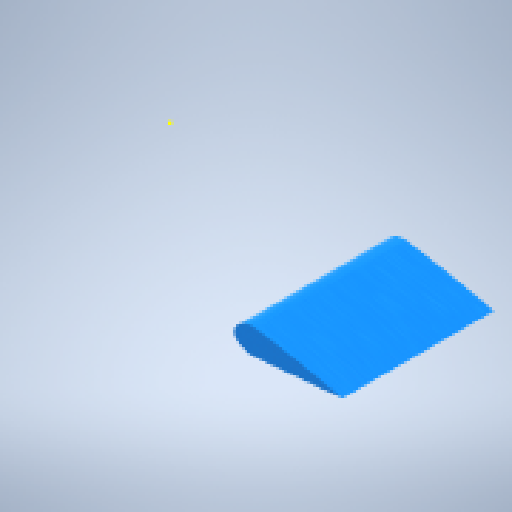
# Autodesk Inventor part: AIL outboard outer foam assembly
Saved by Autodesk Inventor 2025.2 (Build 292293000, 293)
## iProperties
Created: 2024-11-18
Part Number: AIL outboard outer foam assembly
Material: Polyurethane Foam
Document SubType Name: Modeling
Designer: thoma
Density: 0.032 g/cm^3
Appearance: Coarse Textured - Umber
Author: thoma
Autodesk Inventor part; units mm, degrees
ref_plane "YZ Plane" through (0, 0, 0) normal (1, 0, 0) x (0, 1, 0)
ref_plane "XZ Plane" through (0, 0, 0) normal (0, 1, 0) x (-1, 0, 0)
ref_plane "XY Plane" through (0, 0, 0) normal (0, 0, 1) x (1, 0, 0)
sketch "Sketch1" plane through (0, 0, 0) normal (0, 0, 1) x (1, 0, 0)
  spline S0 degree 5 poles (217.3654, -7.5638) (217.3859, -7.562) (219.4778, -7.3868) (223.5726, -7.0416) (229.5629, -6.5311) (237.2988, -5.8637) (246.5067, -5.0508) (255.1715, -4.2808) (263.0989, -3.5455) (270.5088, -2.8843) (276.8391, -2.2398) (282.9867, -1.7375) (287.2724, -1.1764) (292.3303, -0.9034) (294.139, -0.4203) (298.1203, -0.3746) (298.262, -0.0558) (299.6943, -0.05) (299.9984, -0.0244) (300, 0) (300.0016, 0.0244) (299.7036, 0.09) (298.2843, 0.2856) (298.1861, 0.6201) (294.2411, 1.1852) (292.5088, 1.8941) (287.5168, 2.8048) (283.3251, 3.8823) (277.2635, 5.114) (271.0288, 6.4738) (263.7046, 7.9415) (255.8588, 9.4927) (247.2609, 11.1039) (238.144, 12.7436) (230.4968, 14.0478) (224.5814, 15.0163) (220.5538, 15.6564) (218.5257, 15.9738) knots 0.848643 0.848643 0.848643 0.848643 0.848643 0.848643 0.848791 0.863714 0.878289 0.892459 0.906165 0.919343 0.931928 0.943844 0.955007 0.965319 0.974656 0.982848 0.989595 0.994445 1 1 1 1 1 1.005555 1.010406 1.017155 1.025351 1.034694 1.045016 1.056192 1.068127 1.080735 1.093944 1.107687 1.121902 1.13653 1.151213 1.151213 1.151213 1.151213 1.151213 1.151213
  line L0 (200, 103) -> (200, -97) construction
  line L1 (300, -103) -> (300, 103) construction
  line L2 (200, 3.7134) -> (300, 0) construction
  circle A0 centre (225, 2.7851) radius 2.5 construction
  line L3 (205.8741, -8.5266) -> (228.8566, -6.6009) construction
  arc A1 (208.1717, -8.3262) -> (226.5577, -6.7856) centre (-233.8691, 5377.8161) ccw construction
  line L4 (230.0222, 14.1744) -> (207.0292, 17.7732) construction
  arc A2 (227.7165, 14.4952) -> (209.3227, 17.3741) centre (49.5564, -1063.5951) ccw construction
  spline S1 degree 4 poles (217.6716, -7.5381) (213.6705, -8.2359) (189.5382, -3.5576) (201.4741, 15.1863) (214.1486, 16.1309) (218.5257, 15.9738) knots 0 0 0 0 0 0.508217 0.817556 0.817556 0.817556 0.817556 0.817556
  line L5 (212.7843, 16.1798) -> (224.2671, 15.7678) construction
  arc A3 (223.0904, 15.5928) -> (213.9454, 15.921) centre (216.7921, -32.3331) ccw construction
  circle A4 centre (208, 3.4163) radius 2.5
  point P0 (299.5428, 0.1089)
  point P1 (298.1739, 0.4338)
  point P2 (295.9008, 0.9681)
  point P3 (292.7367, 1.7025)
  point P4 (288.6996, 2.6229)
  point P5 (283.8129, 3.7134)
  point P6 (278.1048, 4.9545)
  point P7 (271.6086, 6.3255)
  point P8 (264.3621, 7.8039)
  point P9 (256.4085, 9.3663)
  point P10 (247.7946, 10.9887)
  point P11 (238.572, 12.6468)
  point P12 (228.7959, 14.3166)
  point P13 (207.8235, 17.5944)
  point P14 (237.7638, -5.8185)
  point P15 (247.0398, -5.0019)
  point P16 (255.7236, -4.2234)
  point P17 (263.7597, -3.4905)
  point P18 (271.0965, -2.8098)
  point P19 (277.6872, -2.1882)
  point P20 (283.4889, -1.6323)
  point P21 (288.4641, -1.1487)
  point P22 (292.5804, -0.7434)
  point P23 (295.8102, -0.4221)
  point P24 (298.1328, -0.1887)
  point P25 (299.5323, -0.0474)
  point P26 (217.3654, -7.5638)
  point P27 (206.2647, 13.1249)
  point P28 (218.5257, 15.9738)
  dimension "d17" = 100
  dimension "d22" = 5
  dimension "d23" = 75
  dimension "d30" = 5
  constraints: 12 end point, 7 midpoint, 5 centre point, 3 point on circle, 3 point on line, 2 vertical, 42 other
  measures "d17" distance between parallel lines of L1 L0
  measures "d22" diameter of A0
  measures "d23" distance from line of L1 A0.centre
  measures "d30" diameter of A4
sketch "Sketch3" plane through (0, 0, 0) normal (0, 0, 1) x (1, 0, 0)
  point P0 (0, 0)
sketch "Sketch4" plane through (0, 0, 0) normal (0, 0, 1) x (1, 0, 0)
  point P0 (0, 0)
sketch "Sketch5" plane through (0, 0, 0) normal (0, 0, 1) x (1, 0, 0)
  point P0 (0, 0)
sketch "Sketch6" plane through (0, 0, 0) normal (0, 0, 1) x (1, 0, 0)
  point P0 (0, 0)
sketch "Sketch7" plane through (0, 0, 0) normal (0, 0, 1) x (1, 0, 0)
  point P0 (0, 0)
sketch "Sketch8" plane through (0, 0, 0) normal (0, 0, 1) x (1, 0, 0)
  point P0 (0, 0)
extrude "Extrusion2" add sketch "Sketch1" along normal blind 140.333
body "Solid2"
